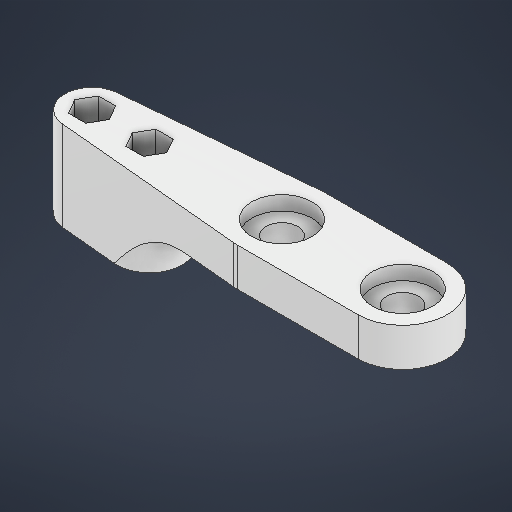
# Autodesk Inventor part: CNC-012-YAxisLimitSwitchMount
Saved by Autodesk Inventor 2026.2 (Build 302298000, 298)
## iProperties
Created: 2026-06-17
Part Number: CNC-012-YAxisLimitSwitchMount
Material: ABS Plastic
Document SubType Name: Modeling
Designer: Kenji
Density: 1.06 g/cm^3
Appearance: Smooth - White
Author: Kenji
Autodesk Inventor part; units mm, degrees
ref_plane "YZ Plane" through (0, 0, 0) normal (1, 0, 0) x (0, 1, 0)
ref_plane "XZ Plane" through (0, 0, 0) normal (0, 1, 0) x (-1, 0, 0)
ref_plane "XY Plane" through (0, 0, 0) normal (0, 0, 1) x (1, 0, 0)
sketch "Sketch1" plane through (0, 0, 0) normal (0, 1, 0) x (-1, 0, 0)
  circle A0 centre (0, 0) radius 1.35
  circle A1 centre (-9.525, 0) radius 1.35
  circle A2 centre (-31.4566, 0) radius 2.63
  circle A3 centre (-51.4566, 0) radius 2.63
  circle A4 centre (0, 0) radius 4.525 construction
  circle A5 centre (-9.525, 0) radius 4.525 construction
  circle A6 centre (-31.4566, 0) radius 7.3925 construction
  circle A7 centre (-51.4566, 0) radius 7.3925 construction
  line L0 (0.412487, 4.50616) -> (-30.782719, 7.361721)
  line L1 (0.412487, -4.50616) -> (-30.782719, -7.361721)
  line L2 (-31.4566, 7.3925) -> (-51.4566, 7.3925)
  line L3 (-31.4566, -7.3925) -> (-51.4566, -7.3925)
  arc A8 (-51.4566, 7.3925) -> (-51.4566, -7.3925) centre (-51.4566, 0) ccw
  arc A9 (-31.4566, -7.3925) -> (-30.782719, -7.361721) centre (-31.4566, 0) ccw
  arc A10 (-30.782719, 7.361721) -> (-31.4566, 7.3925) centre (-31.4566, 0) ccw
  arc A11 (0.412487, -4.50616) -> (0.412487, 4.50616) centre (0, 0) ccw
  dimension "d0" = 2.7
  dimension "d1" = 9.525
  dimension "d2" = 5.26
  dimension "d3" = 21.9316
  dimension "d4" = 20
  dimension "d5" = 3.175
  dimension "d6" = 4.7625
  constraints: 16 point on circle, 12 centre point, 10 tangent, 8 end point, 4 equal radius, 3 coincident, 3 horizontal alignment, 2 concentric, 2 horizontal
  measures "d0" diameter of A0
  measures "d1" distance of point (0, 0) A1.centre
  measures "d2" diameter of A2
  measures "d3" distance of A2.centre A1.centre
  measures "d4" distance of A3.centre A2.centre
  measures "d5" radial gap between concentric circles of A4 A0
  measures "d6" radial gap between concentric circles of A6 A2
extrude "Extrusion1" add sketch "Sketch1" along normal blind 6.35
sketch "Sketch2" plane through (0, 0, 0) normal (0, -1, 0) x (1, 0, 0)
  line L0 (-0.412487, 4.50616) -> (30.782719, 7.361721)
  arc A0 (-0.412487, 4.50616) -> (-0.412487, -4.50616) centre (0, 0) ccw
  line L1 (30.782719, -7.361721) -> (-0.412487, -4.50616)
  arc A1 (30.782719, -7.361721) -> (31.4566, -7.3925) centre (31.4566, 0) ccw
  line L2 (51.4566, -7.3925) -> (31.4566, -7.3925)
  arc A2 (51.4566, -7.3925) -> (51.4566, 7.3925) centre (51.4566, 0) ccw
  line L3 (31.4566, 7.3925) -> (51.4566, 7.3925)
  arc A3 (31.4566, 7.3925) -> (30.782719, 7.361721) centre (31.4566, 0) ccw
  circle A4 centre (0, 0) radius 1.35
  circle A5 centre (51.4566, 0) radius 2.63
  circle A6 centre (31.4566, 0) radius 2.63
  circle A7 centre (9.525, 0) radius 1.35
  circle A8 centre (9.525, 0) radius 5.393274 construction
  line L4 (-0.412487, 4.50616) -> (30.782719, 7.361721)
  arc A9 (9.033364, -5.370819) -> (9.033364, 5.370819) centre (9.525, 0) ccw
  point P0 (9.033364, 5.370819)
  constraints: 4 point on circle, 2 centre point, 2 point on line, 1 coincident, 1 concentric, 1 tangent
extrude "Extrusion2" add sketch "Sketch2" along normal blind 8.5 contours L0 A9 L1 A0
sketch "Sketch3" plane through (0, 6.35, 0) normal (0, 1, 0) x (1, 0, 0)
  circle A0 centre (9.525, 0) radius 1.35
  line L0 (8.095192, -2.4765) -> (6.665384, 0)
  line L1 (6.665384, 0) -> (8.095192, 2.4765)
  line L2 (8.095192, 2.4765) -> (10.954808, 2.4765)
  line L3 (10.954808, 2.4765) -> (12.384616, 0)
  line L4 (12.384616, 0) -> (10.954808, -2.4765)
  line L5 (10.954808, -2.4765) -> (8.095192, -2.4765)
  line L6 (-1.429808, -2.4765) -> (-2.859616, 0)
  line L7 (-2.859616, 0) -> (-1.429808, 2.4765)
  line L8 (-1.429808, 2.4765) -> (1.429808, 2.4765)
  line L9 (1.429808, 2.4765) -> (2.859616, 0)
  line L10 (2.859616, 0) -> (1.429808, -2.4765)
  line L11 (1.429808, -2.4765) -> (-1.429808, -2.4765)
  point P0 (0, 0)
  point P1 (0, 0)
  dimension "d14" = 4.953
  constraints: 24 end point, 2 coincident, 2 horizontal, 1 collinear, 26 other
  measures "d14" distance between parallel lines of L2 L5
extrude "Extrusion3" cut sketch "Sketch3" against normal blind 13.359
fillet "Fillet1" radius 8.5 1 edges at (14.9183, 0, 0)
sketch "Sketch4" plane through (0, 6.35, 0) normal (0, 1, 0) x (1, 0, 0)
  line L0 (1.429808, 2.4765) -> (2.859616, 0)
  line L1 (2.859616, 0) -> (1.429808, -2.4765)
  line L2 (1.429808, -2.4765) -> (-1.429808, -2.4765)
  line L3 (-1.429808, -2.4765) -> (-2.859616, 0)
  line L4 (-2.859616, 0) -> (-1.429808, 2.4765)
  line L5 (-1.429808, 2.4765) -> (1.429808, 2.4765)
  line L6 (10.954808, 2.4765) -> (12.384616, 0)
  line L7 (12.384616, 0) -> (10.954808, -2.4765)
  line L8 (10.954808, -2.4765) -> (8.095192, -2.4765)
  line L9 (8.095192, -2.4765) -> (6.665384, 0)
  line L10 (6.665384, 0) -> (8.095192, 2.4765)
  line L11 (8.095192, 2.4765) -> (10.954808, 2.4765)
  line L12 (-0.412487, -4.50616) -> (30.782719, -7.361721)
  arc A0 (30.782719, -7.361721) -> (31.4566, -7.3925) centre (31.4566, 0) ccw
  line L13 (31.4566, -7.3925) -> (51.4566, -7.3925)
  arc A1 (51.4566, -7.3925) -> (51.4566, 7.3925) centre (51.4566, 0) ccw
  line L14 (51.4566, 7.3925) -> (31.4566, 7.3925)
  arc A2 (31.4566, 7.3925) -> (30.782719, 7.361721) centre (31.4566, 0) ccw
  line L15 (30.782719, 7.361721) -> (-0.412487, 4.50616)
  arc A3 (-0.412487, 4.50616) -> (-0.412487, -4.50616) centre (0, 0) ccw
  circle A4 centre (51.4566, 0) radius 2.63
  circle A5 centre (31.4566, 0) radius 2.63
  circle A6 centre (31.4566, 0) radius 5
  circle A7 centre (51.4566, 0) radius 5
  point P0 (0, 0)
  dimension "d18" = 10
  constraints: 2 centre point, 2 coincident, 1 equal radius
  measures "d18" diameter of A6
extrude "Extrusion4" cut sketch "Sketch4" against normal blind 2.35 contours A6 | A7
body "Solid1"
